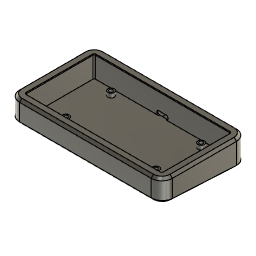
Suffer MFR2 (Autodesk Fusion 360 design; units mm, degrees)
Autodesk Fusion 360 part; units mm, degrees
sketch "PCB Plane" plane through (0, 0, 0) normal (0, 0, 1) x (1, 0, 0)
  line L0 (0, 0) -> (114.3, 0) construction
  line L1 (114.3, 0) -> (114.3, 57.15) construction
  line L2 (114.3, 57.15) -> (0, 57.15) construction
  line L3 (0, 57.15) -> (0, 0) construction
  line L4 (-0.5, -0.5) -> (114.8, -0.5)
  line L5 (114.8, -0.5) -> (114.8, 57.65)
  line L6 (114.8, 57.65) -> (-0.5, 57.65)
  line L7 (-0.5, 57.65) -> (-0.5, -0.5)
  line L8 (-7.5, 64.65) -> (-7.5, -7.5)
  line L9 (-7.5, -7.5) -> (121.8, -7.5)
  line L10 (121.8, -7.5) -> (121.8, 64.65)
  line L11 (121.8, 64.65) -> (-7.5, 64.65)
  dimension "d1" = 114.3
  dimension "d2" = 57.15
  dimension "d3" = 0.5
  dimension "d4" = 7.5
  constraint horizontal L0
  constraint vertical L1
  constraint horizontal L2
  constraint vertical L3
  constraint coincident L0.start L3.end
  measures "d1" distance of L0.start L0.end
  measures "d2" distance of L0.start L2.end
ref_plane "WorkPlane1" through (57.15, 28.575, -3.46) normal (0, 0, 1) x (1, 0, 0)
ref_plane "WorkPlane2" through (57.15, 28.575, 14.6) normal (0, 0, 1) x (1, 0, 0)
extrude "Extrude1" add sketch "PCB Plane" along normal up to surface (14.6 mm away) and the other way up to surface (3.46 mm away)
sketch "Angle Sketch" plane through (121.8, 0, 0) normal (1, 0, 0) x (0, 1, 0)
  line L0 (64.65, 14.6) -> (-7.5, 14.6)
  line L1 (-7.5, 14.6) -> (-7.5, -3.46)
  line L2 (-7.5, -3.46) -> (64.65, -3.46)
  line L3 (64.65, -3.46) -> (64.65, 14.6)
  line L4 (-7.5, 14.6) -> (-7.5, -3.6755)
  line L5 (-7.5, -3.6755) -> (92.363, -8.9091)
  line L6 (-7.5, -3.6755) -> (92.5, -3.6755) construction
  dimension "d11" = 18.2755
  dimension "d12" = 100
  dimension "d13" = 3
  constraint coincident L0.end L1.start
  constraint perpendicular L0 L4
  constraint horizontal L6
  measures "d11" distance of L0.end L4.end
  measures "d12" distance of L4.end L5.end
  measures "d13" angle of L5 L6
ref_plane "WorkPlane3" through (121.8, 42.4315, -6.2923) normal (0, -0.052336, -0.99863) x (0, 0.99863, -0.052336)
sketch "Interior Base Plane" plane through (0, 0, -3.46) normal (0, 0, -1) x (1, 0, 0)
  line L0 (114.8, -57.65) -> (-0.5, -57.65)
  line L1 (-0.5, -57.65) -> (-0.5, 0.5)
  line L2 (-0.5, 0.5) -> (114.8, 0.5)
  line L3 (114.8, 0.5) -> (114.8, -57.65)
  line L4 (-7.5, 7.5) -> (-7.5, -64.65)
  line L5 (-7.5, -64.65) -> (121.8, -64.65)
  line L6 (121.8, -64.65) -> (121.8, 7.5)
  line L7 (121.8, 7.5) -> (-7.5, 7.5)
  line L8 (-7.5, 7.5) -> (121.8, 7.5)
  line L9 (121.8, 7.5) -> (121.8, -64.65)
  line L10 (121.8, -64.65) -> (-7.5, -64.65)
  line L11 (-7.5, -64.65) -> (-7.5, 7.5)
  constraint horizontal L8
  constraint vertical L9
  constraint horizontal L10
  constraint vertical L11
  constraint coincident L5.end L6.start
  constraint coincident L4.start L7.end
extrude "Extrude2" add sketch "Interior Base Plane" along normal up to surface contours L0 L1 L2 L3 | L4 L5 L6 L7 L8 L9 L10 L11 end surface through (121.8, 42.4315, -6.2923) normal (0, -0.052336, -0.99863) offset 0
fillet "Fillet1" radius 9 1 edges at (121.8, -7.5, 5.4623)
fillet "Fillet2" radius 9 1 edges at (121.8, 64.65, 3.5716)
fillet "Fillet3" radius 9 1 edges at (-7.5, 64.65, 3.5716)
fillet "Fillet4" radius 9 1 edges at (-7.5, -7.5, 5.4623)
fillet "Fillet5" radius 1 1 edges at (114.8, 57.65, 5.57)
fillet "Fillet6" radius 1 1 edges at (-0.5, 57.65, 5.57)
fillet "Fillet7" radius 1 1 edges at (114.8, -0.5, 5.57)
fillet "Fillet8" radius 1 1 edges at (-0.5, -0.5, 5.57)
chamfer "Chamfer1" distance 2 angle 45 8 edges at (-7.5, 28.575, 14.6) (-4.864, 62.014, 14.6) (57.15, 64.65, 14.6) (119.164, 62.014, 14.6) (121.8, 28.575, 14.6) (119.164, -4.864, 14.6) (57.15, -7.5, 14.6) (-4.864, -4.864, 14.6)
chamfer "Chamfer2" distance 2 angle 45 8 edges at (-7.5, 28.575, -5.5661) (-4.864, -4.864, -3.8136) (57.15, -7.5, -3.6755) (119.164, -4.864, -3.8136) (121.8, 28.575, -5.5661) (119.164, 62.014, -7.3186) (57.15, 64.65, -7.4567) (-4.864, 62.014, -7.3186)
chamfer "Chamfer3" distance 0.5 angle 45 4 edges at (57.15, 57.65, 14.6) (-0.5, 28.575, 14.6) (57.15, -0.5, 14.6) (114.8, 28.575, 14.6)
extrude "Extrude3" add 1 faces at (75.7, 17.2158, -4.9708) along direction (0, 0.052336, 0.99863) blind 1
ref_plane "WorkPlane4" through (57.15, 28.575, 0) normal (0, 0, 1) x (1, 0, 0)
sketch "USB C Hole Internal" plane through (0, 57.65, 0) normal (0, -1, 0) x (1, 0, 0)
  line L0 (113.8, 14.1) -> (0.5, 14.1)
  line L1 (0.5, -3.46) -> (113.8, -3.46)
  line L2 (53.975, -3.46) -> (60.325, -3.46)
  line L3 (61.875, -1.91) -> (61.875, -1.35)
  line L4 (60.325, 0.2) -> (53.975, 0.2)
  line L5 (52.425, -1.35) -> (52.425, -1.91)
  arc A0 (53.975, 0.2) -> (52.425, -1.35) centre (53.975, -1.35) ccw
  arc A1 (61.875, -1.35) -> (60.325, 0.2) centre (60.325, -1.35) ccw
  arc A2 (60.325, -3.46) -> (61.875, -1.91) centre (60.325, -1.91) ccw
  arc A3 (52.425, -1.91) -> (53.975, -3.46) centre (53.975, -1.91) ccw
  line L6 (0.5, 14.1) -> (0.5, -3.46)
  line L7 (113.8, -3.46) -> (113.8, 14.1)
  line L8 (113.8, -0.2545) -> (114.3, -0.2545)
  line L9 (57.15, 0.2) -> (57.15, -3.46) construction
  dimension "d36" = 1.55
  dimension "d82" = 0.5
  dimension "d83" = 4.725
  dimension "d84" = 57.15
  dimension "d89" = 3.66
  dimension "d90" = 3.66
  constraint horizontal L2
  constraint vertical L3
  constraint horizontal L4
  constraint vertical L5
  constraint tangent L5 A0
  constraint tangent L4 A0
  constraint tangent L4 A1
  constraint tangent L3 A1
  constraint equal A0 A1
  constraint tangent L2 A2
  constraint tangent L3 A2
  constraint equal A0 A2
  constraint tangent L2 A3
  constraint tangent L5 A3
  constraint equal A0 A3
  constraint coincident L7 L8.start
  constraint perpendicular L7 L8
  constraint midpoint L4 L9.start
  constraint midpoint L2 L9.end
  measures "d36" radius of A0
  measures "d82" distance of L8.start L8.end
  measures "d83" distance of L5 L9
  measures "d84" distance of L8.end L9
  measures "d89" distance of L2 L4
  measures "d90" distance of L1 L4
extrude "Extrude4" cut sketch "USB C Hole Internal" against normal through all contours L1 L2 L3 L4 L5 A0 A1 A2 A3
sketch "USB C Hole External" plane through (0, 64.65, 0) normal (0, 1, 0) x (-1, 0, 0)
  line L0 (-60.325, 0.2) -> (-53.975, 0.2)
  arc A0 (-52.425, -1.35) -> (-53.975, 0.2) centre (-53.975, -1.35) ccw
  line L1 (-52.425, -1.35) -> (-52.425, -1.91)
  arc A1 (-53.975, -3.46) -> (-52.425, -1.91) centre (-53.975, -1.91) ccw
  line L2 (-53.975, -3.46) -> (-60.325, -3.46)
  arc A2 (-61.875, -1.91) -> (-60.325, -3.46) centre (-60.325, -1.91) ccw
  line L3 (-61.875, -1.91) -> (-61.875, -1.35)
  arc A3 (-60.325, 0.2) -> (-61.875, -1.35) centre (-60.325, -1.35) ccw
  line L4 (-112.8, -5.4567) -> (-1.5, -5.4567)
  line L5 (-1.5, -5.4567) -> (-1.5, 12.6)
  line L6 (-1.5, 12.6) -> (-112.8, 12.6)
  line L7 (-112.8, 12.6) -> (-112.8, -5.4567)
  line L8 (-52.425, -1.63) -> (-61.875, -1.63) construction
  line L9 (-57.15, 0.2) -> (-57.15, -3.46) construction
  line L10 (-57.65, 2.45) -> (-57.65, -5.71) construction
  line L11 (-190.8318, -1.63) -> (-176.8818, -1.63) construction
  line L12 (-60.325, 2.45) -> (-53.975, 2.45)
  line L13 (-50.175, -1.35) -> (-50.175, -1.91)
  line L14 (-53.975, -5.71) -> (-60.325, -5.71)
  line L15 (-64.125, -1.91) -> (-64.125, -1.35)
  arc A4 (-64.125, -1.91) -> (-60.325, -5.71) centre (-60.325, -1.91) ccw
  arc A5 (-60.325, 2.45) -> (-64.125, -1.35) centre (-60.325, -1.35) ccw
  arc A6 (-50.175, -1.35) -> (-53.975, 2.45) centre (-53.975, -1.35) ccw
  arc A7 (-53.975, -5.71) -> (-50.175, -1.91) centre (-53.975, -1.91) ccw
  dimension "d39" = 8.16
  dimension "d40" = 4.08
  dimension "d42" = 13.95
  dimension "d43" = 3.8
  dimension "d85" = 13.95
  dimension "d86" = 8.16
  dimension "d87" = 6.975
  dimension "d88" = 4.08
  constraint midpoint L1 L8.start
  constraint midpoint L3 L8.end
  constraint midpoint L0 L9.start
  constraint midpoint L2 L9.end
  constraint perpendicular L2 L10
  constraint perpendicular L10 L11
  constraint horizontal L12
  constraint vertical L13
  constraint horizontal L14
  constraint vertical L15
  constraint tangent L14 A4
  constraint tangent L15 A4
  constraint tangent L15 A5
  constraint tangent L12 A5
  constraint equal A4 A5
  constraint tangent L12 A6
  constraint tangent L13 A6
  constraint equal A4 A6
  constraint tangent L13 A7
  constraint tangent L14 A7
  constraint equal A4 A7
  measures "d39" distance of L10.start L10.end
  measures "d40" distance of L8 L10.start
  measures "d42" distance of L11.start L11.end
  measures "d43" radius of A4
  measures "d85" distance of L13 L15
  measures "d86" distance of L12 L14
  measures "d87" distance of L9 L15
  measures "d88" distance of L8.end L14
extrude "Extrude5" cut sketch "USB C Hole External" against normal blind 6.0905 contours L4 L12 L13 L15 A4 A5 A6 A7 | L4 L14 A4 A7
chamfer "Chamfer4" distance 0.25 angle 45 10 edges at (50.8426, 64.65, -4.0613) (63.4574, 64.65, -4.0613) (64.125, 64.65, -1.63) (63.012, 64.65, 1.337) (57.15, 64.65, 2.45) (51.288, 64.65, 1.337) (50.175, 64.65, -1.63) (57.15, 64.3831, -5.71) (61.0187, 64.4504, -5.6461) (53.2813, 64.4504, -5.6461)
sketch "Hole Tops" plane through (0, 0, 0) normal (0, 0, 1) x (1, 0, 0)
  line L0 (0, 0) -> (114.3, 0) construction
  line L1 (114.3, 0) -> (114.3, 57.15) construction
  line L2 (114.3, 57.15) -> (0, 57.15) construction
  line L3 (0, 57.15) -> (0, 0) construction
  circle A0 centre (19.05, 14.2875) radius 2.75
  circle A1 centre (95.25, 14.2875) radius 2.75
  circle A2 centre (95.25, 52.3875) radius 2.75
  circle A3 centre (19.05, 52.3875) radius 2.75
  dimension "d93" = 57.15
  dimension "d94" = 114.3
  dimension "d95" = 5.5
  dimension "d96" = 19.05
  dimension "d97" = 14.2875
  dimension "d98" = 19.05
  dimension "d99" = 14.2875
  dimension "d100" = 4.7625
  dimension "d101" = 19.05
  dimension "d102" = 4.7625
  dimension "d103" = 19.05
  constraint horizontal L0
  constraint vertical L1
  constraint horizontal L2
  constraint vertical L3
  constraint coincident L0.start L3.end
  constraint equal A0 A3
  constraint equal A0 A2
  constraint equal A0 A1
  measures "d93" distance of L0.start L2.end
  measures "d94" distance of L0.start L0.end
  measures "d95" diameter of A0
  measures "d96" distance of L3 A0.centre
  measures "d97" distance of L0 A0.centre
  measures "d98" distance of L1 A1.centre
  measures "d99" distance of L0 A1.centre
  measures "d100" distance of L2 A2.centre
  measures "d101" distance of L1 A2.centre
  measures "d102" distance of L2 A3.centre
  measures "d103" distance of L3 A3.centre
extrude "Extrude6" add sketch "Hole Tops" against normal blind 3.46
hole "Hole5" at (19.05, 52.3875, 0) direction (0, 0, -1) diameter 3.2 depth 4 tip angle 180
hole "Hole6" at (19.05, 14.2875, 0) direction (0, 0, -1) diameter 3.2 depth 4 tip angle 180
hole "Hole7" at (95.25, 52.3875, 0) direction (0, 0, -1) diameter 3.2 depth 4 tip angle 180
hole "Hole8" at (95.25, 14.2875, 0) direction (0, 0, -1) diameter 3.2 depth 4 tip angle 180
sketch "Sketch11" plane through (0, 57.65, 0) normal (0, -1, 0) x (1, 0, 0)
  arc A0 (60.325, -3.46) -> (61.875, -1.91) centre (60.325, -1.91) ccw
  line L0 (60.325, -3.46) -> (113.8, -3.46)
  line L1 (113.8, -3.46) -> (113.8, 14.1)
  line L2 (113.8, 14.1) -> (0.5, 14.1)
  line L3 (0.5, 14.1) -> (0.5, -3.46)
  line L4 (0.5, -3.46) -> (53.975, -3.46)
  arc A1 (52.425, -1.91) -> (53.975, -3.46) centre (53.975, -1.91) ccw
  line L5 (52.425, -1.91) -> (52.425, -1.35)
  arc A2 (53.975, 0.2) -> (52.425, -1.35) centre (53.975, -1.35) ccw
  line L6 (53.975, 0.2) -> (60.325, 0.2)
  arc A3 (61.875, -1.35) -> (60.325, 0.2) centre (60.325, -1.35) ccw
  line L7 (61.875, -1.35) -> (61.875, -1.91)
  line L8 (0.5, -3.46) -> (113.8, -3.46) construction
  line L9 (57.15, -3.46) -> (57.15, 0.2) construction
  line L10 (61.875, 0.2) -> (52.425, 0.2)
  line L11 (52.425, 0.2) -> (52.425, -3.46)
  line L12 (52.425, -3.46) -> (61.875, -3.46)
  line L13 (61.875, -3.46) -> (61.875, 0.2)
  line L14 (61.875, 0.2) -> (52.425, -3.46) construction
  line L15 (52.425, 0.2) -> (61.875, -3.46) construction
  line L16 (62.9565, -3.46) -> (62.9565, 2.3)
  line L17 (51.3435, 2.3) -> (51.3435, -3.46)
  line L18 (51.3435, 2.3) -> (62.9565, 2.3)
  point P0 (57.15, -1.63)
  dimension "d121" = 2.1
  dimension "d122" = 5.8065
  dimension "d123" = 5.8065
  constraint coincident L3.end L4.start
  constraint coincident L0.end L1.start
  constraint midpoint L8 L9.start
  constraint coincident L6 L9.end
  constraint perpendicular L6 L9
  constraint horizontal L10
  constraint perpendicular L10 L11
  constraint parallel L10 L12
  constraint parallel L11 L13
  constraint coincident L14 P0
  constraint coincident L15 P0
  constraint midpoint L9 P0
  constraint perpendicular L16 L18
  measures "d121" distance of L10 L18
  measures "d122" distance of L9 L16
  measures "d123" distance of L9 L17
move_body "Move1" [rolled back] rotate angle -3
equation "d44 = -4.5025 mm - 1.588 mm"
equation "d87 = ( 13.95 / 2 ) * 1 mm"
equation "d88 = ( 8.16 / 2 ) * 1 mm"
equation "d93 = ( 19.05 * 3 ) * 1 mm"
equation "d94 = ( 19.05 * 6 ) * 1 mm"
equation "d97 = ( 19.05 * 0.75 ) * 1 mm"
equation "d99 = ( 0.75 * 19.05 ) * 1 mm"
equation "d100 = 19.05 mm * 0.25"
equation "d102 = 19.05 mm * 0.25"
equation "d121 = 1.6 mm + 0.5 mm"
equation "d122 = ( ( 11.113 + 0.5 ) / 2 ) * 1 mm"
equation "d123 = d122"
